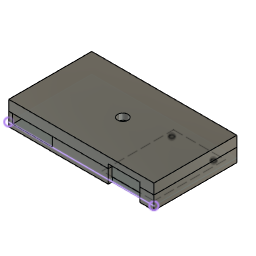
ESP3286 Case (Autodesk Fusion 360 design; units mm, degrees)
Autodesk Fusion 360 part; units mm, degrees
sketch "Sketch1" plane through (0, 0, 0) normal (0, 0, 1) x (1, 0, 0)
  line L0 (0, 0) -> (70, 0)
  line L1 (70, 0) -> (70, 40)
  line L2 (70, 40) -> (0, 40)
  line L3 (0, 40) -> (0, 0)
  dimension "d1" = 70
  dimension "d2" = 40
  constraint horizontal L0
  constraint vertical L1
  constraint horizontal L2
  constraint vertical L3
  constraint coincident L0.start L3.end
  measures "d1" distance of L0.start L0.end
  measures "d2" distance of L0.start L2.end
extrude "Extrude1" add sketch "Sketch1" along normal blind 2 makes body 1
sketch "Sketch2" plane through (0, 0, 2) normal (0, 0, 1) x (-1, 0, 0)
  line L0 (0, -40) -> (0, 0)
  line L1 (0, 0) -> (-70, 0)
  line L2 (-70, 0) -> (-70, -40)
  line L3 (-70, -40) -> (0, -40)
  line L4 (-43, -36.45) -> (-68, -36.45) construction
  line L5 (-68, -36.45) -> (-68, -2.05) construction
  line L6 (-68, -2.05) -> (-43, -2.05) construction
  line L7 (-43, -2.05) -> (-43, -36.45) construction
  circle A0 centre (-65.56, -33.2) radius 0.95
  circle A1 centre (-45.44, -33.2) radius 0.95
  line L8 (0, 0) -> (-70, 0)
  dimension "d5" = 25
  dimension "d6" = 34.4
  dimension "d7" = 2
  dimension "d8" = 1.9
  dimension "d11" = 3.25
  dimension "d12" = 2.44
  dimension "d13" = 1.9
  dimension "d14" = 3.25
  dimension "d15" = 2.44
  dimension "d107" = 2.05
  constraint horizontal L4
  constraint vertical L5
  constraint horizontal L6
  constraint vertical L7
  measures "d5" distance of L4.start L4.end
  measures "d6" distance of L4.start L6.end
  measures "d7" distance of L2 L5
  measures "d8" diameter of A0
  measures "d11" distance of L4 A0.centre
  measures "d12" distance of L5 A0.centre
  measures "d13" diameter of A1
  measures "d14" distance of L4 A1.centre
  measures "d15" distance of L7 A1.centre
  measures "d107" distance of L6 L8
extrude "Extrude2" add sketch "Sketch2" along normal blind 2 contours A1 bodies 1
extrude "Extrude3" add sketch "Sketch2" along normal blind 2 contours A0 bodies 1
sketch "Sketch3" plane through (0, 0, 2) normal (0, 0, 1) x (1, 0, 0)
  line L0 (6, 30) -> (16.5, 30) construction
  line L1 (16.5, 30) -> (16.5, 17.4) construction
  line L2 (16.5, 17.4) -> (6, 17.4) construction
  line L3 (6, 17.4) -> (6, 30) construction
  circle A0 centre (8.5, 27.5) radius 1.5
  dimension "d22" = 10.5
  dimension "d23" = 12.6
  dimension "d24" = 3
  dimension "d25" = 2.5
  dimension "d30" = 2.5
  constraint horizontal L0
  constraint vertical L1
  constraint horizontal L2
  constraint vertical L3
  measures "d22" distance of L0.start L0.end
  measures "d23" distance of L0.start L2.end
  measures "d24" diameter of A0
  measures "d25" distance of L0 A0.centre
  measures "d30" distance of L3 A0.centre
extrude "Extrude4" add sketch "Sketch3" along normal blind 4 bodies 1
sketch "Sketch4" plane through (0, 0, 2) normal (0, 0, 1) x (1, 0, 0)
  line L0 (30, 40) -> (40, 40)
  line L1 (40, 40) -> (40, 10)
  line L2 (40, 10) -> (30, 10)
  line L3 (30, 10) -> (30, 40)
  line L4 (70, 40) -> (0, 40)
  line L5 (0, 40) -> (0, 0) construction
  dimension "d31" = 10
  dimension "d32" = 30
  dimension "d36" = 30
  constraint horizontal L0
  constraint vertical L1
  constraint horizontal L2
  constraint vertical L3
  constraint collinear L0 L4
  measures "d31" distance of L0.start L0.end
  measures "d32" distance of L0.start L2.end
  measures "d36" distance of L3 L5
extrude "Extrude5" add sketch "Sketch4" along normal blind 4.46 bodies 1
sketch "Sketch5" plane through (0, 0, 6.46) normal (0, 0, 1) x (-1, 0, 0)
  line L0 (-30, -10) -> (-40, -10)
  line L1 (-40, -10) -> (-40, -40)
  line L2 (-40, -40) -> (-30, -40)
  line L3 (-30, -40) -> (-30, -10)
  circle A0 centre (-35, -20) radius 1.5
  line L4 (-70, -40) -> (0, -40)
  line L5 (-35, -20) -> (-30, -20)
  dimension "d35" = 20
  dimension "d37" = 5
  dimension "d38" = 3
  constraint coincident A0.centre L5.start
  constraint coincident L3 L5.end
  constraint perpendicular L3 L5
  measures "d35" distance of A0.centre L4
  measures "d37" distance of A0.centre L5.end
  measures "d38" diameter of A0
extrude "Extrude6" cut sketch "Sketch5" against normal blind 13 contours A0 bodies 1
sketch "Sketch6" plane through (0, 0, 2) normal (0, 0, 1) x (1, 0, 0)
sketch "Sketch7" plane through (0, 0, 2) normal (0, 0, 1) x (1, 0, 0)
  line L0 (70, 40) -> (68.2, 40)
  line L1 (68.2, 40) -> (68.2, 0)
  line L2 (68.2, 0) -> (70, 0)
  line L3 (70, 0) -> (70, 40)
  line L4 (0, 0) -> (70, 0)
  point P0 (70, 40)
  dimension "d42" = 1.8
  constraint horizontal L0
  constraint vertical L1
  constraint horizontal L2
  constraint vertical L3
  constraint coincident P0 L0.start
  constraint collinear L2 L4
  measures "d42" distance of P0 L0.end
extrude "Extrude7" add sketch "Sketch7" along normal blind 4.46 bodies 1
sketch "Sketch8" plane through (0, 0, 2) normal (0, 0, 1) x (1, 0, 0)
  line L0 (0, 40) -> (1.8, 40)
  line L1 (1.8, 40) -> (1.8, 0)
  line L2 (1.8, 0) -> (0, 0)
  line L3 (0, 0) -> (0, 40)
  line L4 (0, 0) -> (70, 0)
  point P0 (0, 40)
  dimension "d45" = 1.8
  constraint horizontal L0
  constraint vertical L1
  constraint horizontal L2
  constraint vertical L3
  constraint coincident P0 L0.start
  constraint collinear L2 L4
  measures "d45" distance of P0 L0.end
extrude "Extrude8" add sketch "Sketch8" along normal blind 4.46 bodies 1
sketch "Sketch9" plane through (0, 0, 2) normal (0, 0, 1) x (1, 0, 0)
  line L0 (40, 0) -> (21, 0)
  line L1 (21, 0) -> (21, 1.8)
  line L2 (21, 1.8) -> (40, 1.8)
  line L3 (40, 1.8) -> (40, 0)
  line L4 (0, 0) -> (70, 0)
  line L5 (43, 2.05) -> (43, 36.45)
  line L6 (16.5, 17.4) -> (16.5, 0) construction
  point P0 (16.5, 17.4)
  dimension "d48" = 1.8
  dimension "d49" = 3
  dimension "d52" = 4.5
  constraint horizontal L0
  constraint vertical L1
  constraint horizontal L2
  constraint vertical L3
  constraint coincident L0.start L4
  constraint vertical L6
  constraint coincident P0 L6.start
  constraint coincident L4 L6.end
  measures "d48" distance of L0.start L2.end
  measures "d49" distance of L3 L5
  measures "d52" distance of L1 L6
extrude "Extrude9" add sketch "Sketch9" along normal blind 4.46 bodies 1
sketch "Sketch10" plane through (0, 0, 2) normal (0, 0, 1) x (1, 0, 0)
  line L0 (30, 40) -> (21, 40)
  line L1 (21, 40) -> (21, 38.2)
  line L2 (21, 38.2) -> (30, 38.2)
  line L3 (30, 38.2) -> (30, 40)
  line L4 (70, 40) -> (0, 40)
  line L5 (30, 10) -> (30, 40)
  dimension "d53" = 9
  dimension "d54" = 1.8
  constraint horizontal L0
  constraint vertical L1
  constraint horizontal L2
  constraint vertical L3
  constraint coincident L0.start L4
  constraint collinear L3 L5
  measures "d53" distance of L0.start L0.end
  measures "d54" distance of L0.start L2.end
chamfer "Chamfer4" distance 0.5 angle 45 1 edges at (7.1015, 26.9576, 6) on bodies 1
sketch "Sketch11" plane through (0, 0, 2) normal (0, 0, 1) x (1, 0, 0)
  line L0 (16.5, 30) -> (18.3, 30)
  line L1 (18.3, 30) -> (18.3, 17.4)
  line L2 (18.3, 17.4) -> (16.5, 17.4)
  line L3 (16.5, 17.4) -> (16.5, 30)
  point P0 (16.5, 30)
  dimension "d56" = 1.8
  constraint horizontal L0
  constraint vertical L1
  constraint horizontal L2
  constraint vertical L3
  constraint coincident P0 L0.start
  measures "d56" distance of P0 L0.end
extrude "Extrude10" add sketch "Sketch11" along normal blind 4.46 bodies 1
extrude "Extrude11" add sketch "Sketch10" along normal blind 4.46 bodies 1
sketch "Sketch12" plane through (0, 0, 6.46) normal (0, 0, 1) x (-1, 0, 0)
  circle A0 centre (-35, -20) radius 1.5
  line L0 (-40, -40) -> (-21, -40)
  line L1 (-21, -40) -> (-21, -38.2)
  line L2 (-21, -38.2) -> (-30, -38.2)
  line L3 (-30, -38.2) -> (-30, -10)
  line L4 (-30, -10) -> (-40, -10)
  line L5 (-40, -10) -> (-40, -40)
  line L6 (-37, -40) -> (-33, -40)
  line L7 (-33, -40) -> (-33, -38)
  line L8 (-33, -38) -> (-37, -38)
  line L9 (-37, -38) -> (-37, -40)
  dimension "d61" = 4
  dimension "d62" = 2
  dimension "d63" = 3
  constraint horizontal L6
  constraint vertical L7
  constraint horizontal L8
  constraint vertical L9
  constraint coincident L0 L6.start
  measures "d61" distance of L6.start L6.end
  measures "d62" distance of L6.start L8.end
  measures "d63" distance of L5 L9
extrude "Extrude12" cut sketch "Sketch12" against normal blind 4 contours L0 L6 L7 L8 L9 bodies 1
sketch "Sketch13" plane through (0, 0, 2) normal (0, 0, 1) x (-1, 0, 0)
  line L0 (0, 15) -> (-70, 15)
  line L1 (-70, 15) -> (-70, 55)
  line L2 (-70, 55) -> (0, 55)
  line L3 (0, 55) -> (0, 15)
  dimension "d66" = 40
  dimension "d67" = 70
  constraint horizontal L0
  constraint vertical L1
  constraint horizontal L2
  constraint vertical L3
  measures "d66" distance of L0.end L1.end
  measures "d67" distance of L0.start L0.end
extrude "Extrude13" add sketch "Sketch13" along normal blind 5 separate body makes body 2
sketch "Sketch15" plane through (0, 0, 2) normal (0, 0, -1) x (1, 0, 0)
  line L0 (70, 55) -> (0, 55)
  line L1 (0, 55) -> (0, 15)
  line L2 (0, 15) -> (70, 15)
  line L3 (70, 15) -> (70, 55)
  line L4 (36.975, 15) -> (33.025, 15)
  line L5 (33.025, 15) -> (33.025, 17)
  line L6 (33.025, 17) -> (36.975, 17)
  line L7 (36.975, 17) -> (36.975, 15)
  line L8 (36.975, 17) -> (70, 17) construction
  line L9 (33.025, 17) -> (0, 17) construction
  dimension "d73" = 3.95
  dimension "d74" = 2
  constraint horizontal L4
  constraint vertical L5
  constraint horizontal L6
  constraint vertical L7
  constraint coincident L2 L4.start
  constraint coincident L3 L8.end
  constraint perpendicular L3 L8
  constraint coincident L1 L9.end
  constraint perpendicular L1 L9
  constraint equal L8 L9
  measures "d73" distance of L4.start L4.end
  measures "d74" distance of L4.start L6.end
extrude "Extrude15" add sketch "Sketch15" along normal blind 3.5 contours L2 L4 L5 L6 L7 bodies 2
chamfer "Chamfer5" distance 0.5 angle 45 1 edges at (33.025, -16, -1.5) on bodies 2
chamfer "Chamfer6" distance 0.5 angle 45 1 edges at (36.975, -16, -1.5) on bodies 2
copy_body "Body->Comp1" bodies 1 removing the originals makes body 3 in component "Rückseite"
copy_body "Body->Comp2" bodies 2 removing the originals makes body 4 in component "Deckel"
sketch "Sketch16" plane through (0, 0, 11.46) normal (0, 0, 1) x (-1, 0, 0)
  line L0 (0, 0) -> (-70, 0)
  line L1 (-70, 0) -> (-70, -40)
  line L2 (-70, -40) -> (0, -40)
  line L3 (0, -40) -> (0, 0)
  line L4 (0, -40) -> (-70, 0) construction
  line L5 (-70, -40) -> (0, 0) construction
  circle A0 centre (-35, -20) radius 2.5
  dimension "d83" = 5
  constraint coincident L2.end L3.start
  constraint coincident L0.end L1.start
  constraint coincident L1.end L2.start
  constraint coincident L0.start L3.end
  constraint midpoint L5 A0.centre
  measures "d83" diameter of A0
extrude "Extrude1'" cut sketch "Sketch16" against normal blind 3 contours A0 sketch seen with x (1, 0, 0) y (0, 1, 0) z (0, 0, 1) at (0, -55, -4.46) bodies 4 in component "Deckel"
sketch "Sketch17" plane through (0, 0, 8.46) normal (0, 0, 1) x (-1, 0, 0)
  circle A0 centre (-35, -20) radius 2.5
  circle A1 centre (-35, -20) radius 1.5
  dimension "d86" = 3
  constraint concentric A0 A1
  measures "d86" diameter of A1
extrude "Extrude2'" cut sketch "Sketch17" against normal blind 2 contours A1 sketch seen with x (1, 0, 0) y (0, 1, 0) z (0, 0, 1) at (0, -55, -4.46) bodies 4 in component "Deckel"
delete_face "DeleteFace1" 1 faces at (7.3983, 26.7489, 5.6667) on bodies 3 in component "Rückseite"
extrude "Extrude1''" add 1 faces at (8.03, 27.9662, 6) along direction (0, 0, 1) blind 0.4 on bodies 3 bodies 3 in component "Rückseite"
extrude "Extrude2''" add 1 faces at (45.5983, 32.9258, 4) along direction (0, 0, 1) blind 2.4 on bodies 3 bodies 3 in component "Rückseite"
extrude "Extrude3'" add 1 faces at (65.3279, 33.4154, 4) along direction (0, 0, 1) blind 2.4 on bodies 3 bodies 3 in component "Rückseite"
sketch "Sketch18" plane through (0, 40, 0) normal (0, 1, 0) x (-1, 0, 0)
  line L0 (-37, 2.46) -> (-37, 6.46)
  line L1 (-37, 6.46) -> (-40, 6.46)
  line L2 (-40, 6.46) -> (-40, 2)
  line L3 (-40, 2) -> (-68.2, 2)
  line L4 (-68.2, 2) -> (-68.2, 6.46)
  line L5 (-68.2, 6.46) -> (-70, 6.46)
  line L6 (-70, 6.46) -> (-70, 0)
  line L7 (-70, 0) -> (0, 0)
  line L8 (0, 0) -> (0, 6.46)
  line L9 (0, 6.46) -> (-1.8, 6.46)
  line L10 (-1.8, 6.46) -> (-1.8, 2)
  line L11 (-1.8, 2) -> (-21, 2)
  line L12 (-21, 2) -> (-21, 6.46)
  line L13 (-21, 6.46) -> (-33, 6.46)
  line L14 (-33, 6.46) -> (-33, 2.46)
  line L15 (-33, 2.46) -> (-37, 2.46)
  line L16 (-37.5, 0) -> (-32.5, 0)
  line L17 (-32.5, 0) -> (-32.5, 1)
  line L18 (-32.5, 1) -> (-37.5, 1)
  line L19 (-37.5, 1) -> (-37.5, 0)
  line L20 (-32.5, 0) -> (0, 0) construction
  line L21 (-37.5, 0) -> (-70, 0) construction
  dimension "d95" = 5
  dimension "d96" = 1
  constraint horizontal L16
  constraint vertical L17
  constraint horizontal L18
  constraint vertical L19
  constraint coincident L7 L16.start
  constraint coincident L7.end L8.start
  constraint perpendicular L8 L20
  constraint coincident L6.end L7.start
  constraint perpendicular L6 L21
  constraint equal L20 L21
  measures "d95" distance of L16.start L16.end
  measures "d96" distance of L16.start L18.end
extrude "Extrude4'" add sketch "Sketch18" along normal blind 5 contours L7 L16 L17 L18 L19 bodies 3 in component "Rückseite"
fillet "Fillet1" radius 2.5 1 edges at (37.5, 45, 0.5) on bodies 3 in component "Rückseite"
fillet "Fillet2" radius 2.5 1 edges at (32.5, 45, 0.5) on bodies 3 in component "Rückseite"
sketch "Sketch19" plane through (0, 0, 1) normal (0, 0, 1) x (-1, 0, 0)
  arc A0 (-37.5, -42.5) -> (-32.5, -42.5) centre (-35, -42.5) ccw
  line L0 (-32.5, -42.5) -> (-32.5, -40)
  line L1 (-32.5, -40) -> (-37.5, -40)
  line L2 (-37.5, -40) -> (-37.5, -42.5)
  line L3 (-32.5, -42.5) -> (-37.5, -42.5) construction
  line L4 (-35, -42.5) -> (-35, -45) construction
  circle A1 centre (-35, -42.5) radius 0.75
  dimension "d103" = 1.5
  constraint coincident A0.end L0.start
  constraint coincident A0.start L2.end
  constraint coincident A0.centre L4.start
  constraint midpoint A0 L4.end
  measures "d103" diameter of A1
extrude "Extrude5'" cut sketch "Sketch19" against normal blind 1 contours A1 bodies 3 in component "Rückseite"
chamfer "Chamfer1" distance 0.5 angle 45 1 edges at (35.6992, 42.2288, 1) on bodies 3 in component "Rückseite"
sketch "Sketch20" plane through (68.2, 0, 0) normal (-1, 0, 0) x (0, -1, 0)
  line L0 (-40, 2) -> (0, 2)
  line L1 (0, 2) -> (0, 6.46)
  line L2 (0, 6.46) -> (-40, 6.46)
  line L3 (-40, 6.46) -> (-40, 2)
  line L4 (0, 2) -> (-2, 2)
  line L5 (-2, 2) -> (-2, 6.46)
  line L6 (-2, 6.46) -> (0, 6.46)
  line L7 (0, 6.46) -> (0, 2)
  dimension "d108" = 2
  dimension "d109" = 4.46
  constraint horizontal L4
  constraint vertical L5
  constraint horizontal L6
  constraint vertical L7
  constraint coincident L0.end L1.start
  measures "d108" distance of L0.end L4.end
  measures "d109" distance of L0.end L1.end
extrude "Extrude6'" add sketch "Sketch20" along normal blind 5 contours L0 L1 L2 L4 L5 L6 L7 bodies 3 in component "Rückseite"
extrude "Extrude7'" add 1 faces at (40, 1.2, 3.4867) along direction (1, 0, 0) blind 8 on bodies 3 bodies 3 in component "Rückseite"
sketch "Sketch21" plane through (0, 0, 2) normal (0, 0, 1) x (1, 0, 0)
  line L0 (68.2, 36.7) -> (68.2, 40)
  line L1 (43, 40) -> (43, 36.7)
  line L2 (43, 36.45) -> (68, 36.45)
  line L3 (68.2, 2) -> (68.2, 40)
  line L4 (50.6, 36.7) -> (50.6, 40)
  line L5 (60.6, 40) -> (60.6, 36.7)
  line L6 (50.6, 38.35) -> (43, 38.35) construction
  line L7 (60.6, 38.35) -> (68.2, 38.35) construction
  line L8 (43, 36.7) -> (50.6, 36.7)
  line L9 (60.6, 36.7) -> (68.2, 36.7)
  line L10 (68.2, 40) -> (60.6, 40)
  line L11 (50.6, 40) -> (43, 40)
  line L12 (70, 40) -> (0, 40) construction
  dimension "d114" = 25.2
  dimension "d116" = 0.25
  dimension "d117" = 10
  constraint horizontal L8
  constraint vertical L0
  constraint horizontal L10
  constraint vertical L1
  constraint collinear L0 L3
  constraint vertical L4
  constraint vertical L5
  constraint coincident L5.end L8
  constraint midpoint L4 L6.start
  constraint midpoint L1 L6.end
  constraint midpoint L5 L7.start
  constraint midpoint L0 L7.end
  constraint equal L6 L7
  constraint collinear L8 L9
  constraint collinear L10 L11
  constraint collinear L11 L12
  measures "d114" distance of L1.end L0.start
  measures "d116" distance of L2 L8
  measures "d117" distance of L5.end L4.start
extrude "Extrude8'" add sketch "Sketch21" along normal blind 4.46 bodies 3 in component "Rückseite"
extrude "Extrude9'" add 1 faces at (43, 38.9, 3.4867) along direction (-1, 0, 0) blind 3 on bodies 3 bodies 3 in component "Rückseite"
extrude "Extrude10'" add 1 faces at (40, 27.8, 3.4867) along direction (1, 0, 0) blind 2.5 on bodies 3 bodies 3 in component "Rückseite"
sketch "Sketch22" plane through (0, 0, 0) normal (0, -1, 0) x (1, 0, 0)
  line L0 (0, 6.46) -> (70, 6.46)
  line L1 (70, 6.46) -> (70, 11.46)
  line L2 (70, 11.46) -> (0, 11.46)
  line L3 (0, 11.46) -> (0, 6.46)
  line L4 (48, 6.46) -> (63.2, 6.46)
  line L5 (63.2, 6.46) -> (63.2, 8.46)
  line L6 (63.2, 8.46) -> (48, 8.46)
  line L7 (48, 8.46) -> (48, 6.46)
  point P0 (48, 6.46)
  dimension "d124" = 15.2
  dimension "d125" = 2
  constraint horizontal L4
  constraint vertical L5
  constraint horizontal L6
  constraint vertical L7
  constraint coincident P0 L4.start
  measures "d124" distance of P0 L4.end
  measures "d125" distance of P0 L6.end
extrude "Extrude3''" cut sketch "Sketch22" against normal blind 2 contours L0 L4 L5 L6 L7 sketch seen with x (1, 0, 0) y (0, 1, 0) z (0, 0, 1) at (0, -55, -4.46) bodies 4 in component "Deckel"
sketch "Sketch23" plane through (0, 0, 0) normal (0, -1, 0) x (1, 0, 0)
  line L0 (0, 0) -> (70, 0)
  line L1 (70, 0) -> (70, 6.46)
  line L2 (70, 6.46) -> (63.2, 6.46)
  line L3 (63.2, 6.46) -> (63.2, 2)
  line L4 (63.2, 2) -> (48, 2)
  line L5 (48, 2) -> (48, 6.46)
  line L6 (48, 6.46) -> (21, 6.46)
  line L7 (21, 6.46) -> (21, 2)
  line L8 (21, 2) -> (1.8, 2)
  line L9 (1.8, 2) -> (1.8, 6.46)
  line L10 (1.8, 6.46) -> (0, 6.46)
  line L11 (0, 6.46) -> (0, 0)
  line L12 (48, 2) -> (63.2, 2)
  line L13 (63.2, 2) -> (63.2, 0)
  line L14 (63.2, 0) -> (48, 0)
  line L15 (48, 0) -> (48, 2)
  constraint horizontal L12
  constraint vertical L13
  constraint horizontal L14
  constraint vertical L15
  constraint coincident L0 L13.end
  constraint coincident L4.end L5.start
extrude "Extrude11'" cut sketch "Sketch23" against normal blind 2 contours L0 L4 L12 L13 L14 L15 bodies 3 in component "Rückseite"
component "Rückseite" placed x (1, 0, 0) y (0, 1, 0) z (0, 0, 1) at (0, 0, 0)
component "Deckel" placed x (1, 0, 0) y (0, 1, 0) z (0, 0, 1) at (0, 55, 4.46)
equation "d11 = 1 mm + 2.25 mm"
equation "d12 = 1 mm + 1.44 mm"
equation "d14 = d11"
equation "d15 = d12"
equation "d25 = 1.5 mm + 1 mm"
equation "d30 = 1.5 mm + 1 mm"
equation "d33 = hight"
equation "hight = 4.46 mm"
equation "d43 = hight"
equation "d46 = hight"
equation "d50 = hight"
equation "d57 = hight"
equation "d59 = hight"
equation "d109 = hight"
equation "d118 = hight"
